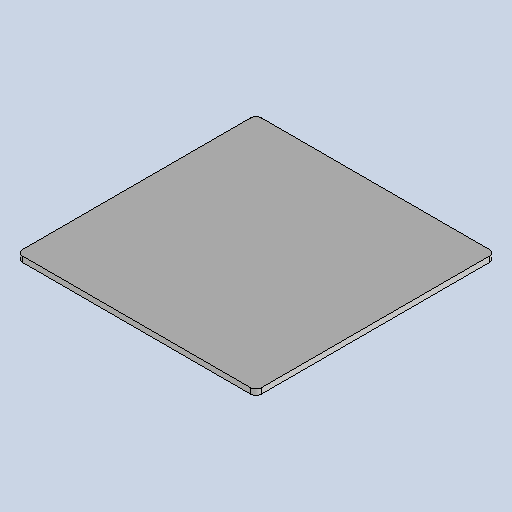
# Autodesk Inventor part: PRS 1200-511 FDS 1000 CUP 1
Saved by Autodesk Inventor 2025.3 (Build 293356030, 356C)
## iProperties
Created: 2025-06-24
Part Number: PRS 1200-511 FDS 1000 CUP 1
Material: Stainless Steel
Document SubType Name: Sheet Metal
Designer: admin
Mass: 118.281 g
Surface Area: 154.663 cm^2
Volume: 14.7851 cm^3
Density: 8 g/cm^3
Flat Pattern Width: 8.6 cm
Flat Pattern Length: 8.6 cm
Flat Pattern Area: 73.96 cm^2
Sheet Metal Rule: AISI304 2mm Die16
Sheet Metal Width: 86,000 mm
Sheet Metal Length: 86,000 mm
Sheet Metal Area: 7396,000 mm^2
Appearance: Default
Author: user
Autodesk Inventor part; units mm, degrees
ref_plane "YZ Plane" through (0, 0, 0) normal (1, 0, 0) x (0, 1, 0)
ref_plane "XZ Plane" through (0, 0, 0) normal (0, 1, 0) x (-1, 0, 0)
ref_plane "XY Plane" through (0, 0, 0) normal (0, 0, 1) x (1, 0, 0)
sketch "Sketch1" plane through (0, 0, 0) normal (0, 0, 1) x (1, 0, 0)
  line L0 (-43, -43) -> (43, -43)
  line L1 (43, -43) -> (43, 43)
  line L2 (43, 43) -> (-43, 43)
  line L3 (-43, 43) -> (-43, -43)
  line L4 (-43, -43) -> (43, 43) construction
  line L5 (43, -43) -> (-43, 43) construction
  point P0 (0, 0)
  dimension "d154" = 86
  dimension "d155" = 86
  measures "d154" distance of L1.end L2.end
  measures "d155" distance of L0.end L1.end
extrude "Plate5" add sketch "Sketch1" along normal blind 2
fillet "Corner Round1" radius 2 4 edges at (43, 43, 1) (-43, 43, 1) (-43, -43, 1) (43, -43, 1)
body "Solid3"
